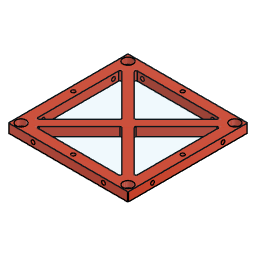
top-holder (Autodesk Fusion 360 design; units mm, degrees)
Autodesk Fusion 360 part; units mm, degrees
sketch "Sketch1" plane through (0, 0, 0) normal (0, 0, 1) x (1, 0, 0)
  line L0 (-44.9, 45) -> (49.5, 45)
  line L1 (49.8, 44.7) -> (49.8, -49.7)
  line L2 (49.5, -50) -> (-44.9, -50)
  line L3 (-45.2, -49.7) -> (-45.2, 44.7)
  arc A0 (-44.9, 45) -> (-45.2, 44.7) centre (-44.9, 44.7) ccw
  arc A1 (49.8, 44.7) -> (49.5, 45) centre (49.5, 44.7) ccw
  arc A2 (49.5, -50) -> (49.8, -49.7) centre (49.5, -49.7) ccw
  arc A3 (-45.2, -49.7) -> (-44.9, -50) centre (-44.9, -49.7) ccw
  point P0 (-45.2, 45)
  point P1 (49.8, 45)
  point P2 (-45.2, -50)
  dimension "d1" = 95
  dimension "d2" = 95
  dimension "d3" = 0.3
  dimension "d4" = 0.3
  constraint horizontal L0
  constraint vertical L1
  constraint horizontal L2
  constraint vertical L3
  constraint coincident P0 L0
  constraint coincident P0 L3
  constraint tangent L0 A0
  constraint tangent L3 A0
  constraint coincident P1 L0
  constraint coincident P1 L1
  constraint tangent L0 A1
  constraint tangent L1 A1
  constraint tangent L1 A2
  constraint tangent L2 A2
  constraint equal A1 A2
  constraint coincident P2 L2
  constraint coincident P2 L3
  constraint tangent L2 A3
  constraint tangent L3 A3
  constraint equal A1 A3
  measures "d1" distance of P0 P1
  measures "d2" distance of P0 P2
  measures "d3" radius of A0
  measures "d4" radius of A1
extrude "Extrude1" add sketch "Sketch1" along normal blind 7
sketch "Sketch2" plane through (0, 0, 7) normal (0, 0, 1) x (-1, 0, 0)
  arc A0 (44.9, -45) -> (45.2, -44.7) centre (44.9, -44.7) ccw
  line L0 (45.2, -44.7) -> (45.2, 49.7)
  arc A1 (45.2, 49.7) -> (44.9, 50) centre (44.9, 49.7) ccw
  line L1 (44.9, 50) -> (-49.5, 50)
  arc A2 (-49.5, 50) -> (-49.8, 49.7) centre (-49.5, 49.7) ccw
  line L2 (-49.8, 49.7) -> (-49.8, -44.7)
  arc A3 (-49.8, -44.7) -> (-49.5, -45) centre (-49.5, -44.7) ccw
  line L3 (-49.5, -45) -> (44.9, -45)
  line L4 (-38.8, 42) -> (34.2, 42)
  line L5 (37.2, 39) -> (37.2, -34)
  line L6 (34.2, -37) -> (-38.8, -37)
  line L7 (-41.8, -34) -> (-41.8, 39)
  arc A4 (-41.8, -34) -> (-38.8, -37) centre (-38.8, -34) ccw
  arc A5 (-38.8, 42) -> (-41.8, 39) centre (-38.8, 39) ccw
  arc A6 (37.2, 39) -> (34.2, 42) centre (34.2, 39) ccw
  arc A7 (34.2, -37) -> (37.2, -34) centre (34.2, -34) ccw
  point P0 (-41.8, 42)
  point P1 (37.2, 42)
  point P2 (-41.8, -37)
  dimension "d7" = 79
  dimension "d8" = 79
  dimension "d9" = 8
  dimension "d10" = 8
  dimension "d11" = 3
  constraint horizontal L4
  constraint vertical L5
  constraint horizontal L6
  constraint vertical L7
  constraint coincident P2 L6
  constraint coincident P2 L7
  constraint tangent L6 A4
  constraint tangent L7 A4
  constraint coincident P0 L4
  constraint coincident P0 L7
  constraint tangent L4 A5
  constraint tangent L7 A5
  constraint equal A4 A5
  constraint coincident P1 L4
  constraint coincident P1 L5
  constraint tangent L4 A6
  constraint tangent L5 A6
  constraint equal A4 A6
  constraint tangent L5 A7
  constraint tangent L6 A7
  constraint equal A4 A7
  measures "d7" distance of P0 P1
  measures "d8" distance of P0 P2
  measures "d9" distance of L1 L4
  measures "d10" distance of L2 L7
  measures "d11" radius of A4
extrude "Extrude2" cut sketch "Sketch2" against normal blind 10 contours L4 L5 L6 L7 A4 A5 A6 A7
sketch "Sketch3" plane through (0, 0, 7) normal (0, 0, 1) x (-1, 0, 0)
  line L0 (34.2, -37) -> (-38.8, -37)
  arc A0 (-41.8, -34) -> (-38.8, -37) centre (-38.8, -34) ccw
  line L1 (-41.8, -34) -> (-41.8, 39)
  arc A1 (-38.8, 42) -> (-41.8, 39) centre (-38.8, 39) ccw
  line L2 (-38.8, 42) -> (34.2, 42)
  arc A2 (37.2, 39) -> (34.2, 42) centre (34.2, 39) ccw
  line L3 (37.2, 39) -> (37.2, -34)
  arc A3 (34.2, -37) -> (37.2, -34) centre (34.2, -34) ccw
  arc A4 (44.9, -45) -> (45.2, -44.7) centre (44.9, -44.7) ccw
  line L4 (45.2, -44.7) -> (45.2, 49.7)
  arc A5 (45.2, 49.7) -> (44.9, 50) centre (44.9, 49.7) ccw
  line L5 (44.9, 50) -> (-49.5, 50)
  arc A6 (-49.5, 50) -> (-49.8, 49.7) centre (-49.5, 49.7) ccw
  line L6 (-49.8, 49.7) -> (-49.8, -44.7)
  arc A7 (-49.8, -44.7) -> (-49.5, -45) centre (-49.5, -44.7) ccw
  line L7 (-49.5, -45) -> (44.9, -45)
  line L8 (45.2, -45) -> (-49.75, 49.95)
sketch "Sketch4" plane through (0, 0, 7) normal (0, 0, 1) x (-1, 0, 0)
  line L0 (45.2, 50) -> (-49.8, -45)
sketch "Sketch5" plane through (0, 0, 7) normal (0, 0, 1) x (-1, 0, 0)
  line L0 (40.0749, -34.9251) -> (35.1251, -39.8749)
  line L1 (35.1251, -39.8749) -> (-45.1249, 40.3751)
  line L2 (-45.1249, 40.3751) -> (-40.1751, 45.3249)
  line L3 (-40.1751, 45.3249) -> (40.0749, -34.9251)
  line L4 (45.2, -45) -> (-49.75, 49.95)
  dimension "d14" = 3.5
  dimension "d15" = 3.5
  constraint perpendicular L0 L1
  constraint parallel L0 L2
  constraint parallel L1 L3
  measures "d14" distance of L1 L4
  measures "d15" distance of L3 L4
extrude "Extrude3" add sketch "Sketch5" against normal blind 7
sketch "Sketch6" plane through (0, 0, 7) normal (0, 0, 1) x (-1, 0, 0)
  line L0 (35.1251, 44.8749) -> (40.0749, 39.9251)
  line L1 (40.0749, 39.9251) -> (-41.1751, -41.3249)
  line L2 (-41.1751, -41.3249) -> (-46.1249, -36.3751)
  line L3 (-46.1249, -36.3751) -> (35.1251, 44.8749)
  line L4 (45.2, 50) -> (-49.8, -45)
  dimension "d18" = 3.5
  dimension "d19" = 3.5
  constraint perpendicular L0 L1
  constraint parallel L0 L2
  constraint parallel L1 L3
  measures "d18" distance of L3 L4
  measures "d19" distance of L1 L4
extrude "Extrude4" add sketch "Sketch6" against normal blind 7
sketch "Sketch7" plane through (0, 0, 7) normal (0, 0, 1) x (-1, 0, 0)
  line L0 (37.2, 37.0503) -> (37.2, -32.0503)
  line L1 (37.2, -32.0503) -> (2.6497, 2.5)
  line L2 (2.6497, 2.5) -> (37.2, 37.0503)
  line L3 (-2.3, -2.4497) -> (32.2503, -37)
  line L4 (32.2503, -37) -> (-36.8503, -37)
  line L5 (-36.8503, -37) -> (-2.3, -2.4497)
  line L6 (-7.2497, 2.5) -> (-41.8, -32.0503)
  line L7 (-41.8, -32.0503) -> (-41.8, 37.0503)
  line L8 (-41.8, 37.0503) -> (-7.2497, 2.5)
  line L9 (32.2503, 42) -> (-2.3, 7.4497)
  line L10 (-2.3, 7.4497) -> (-36.8503, 42)
  line L11 (-36.8503, 42) -> (32.2503, 42)
  arc A0 (44.9, -45) -> (45.2, -44.7) centre (44.9, -44.7) ccw
  line L12 (45.2, -44.7) -> (45.2, 49.7)
  arc A1 (45.2, 49.7) -> (44.9, 50) centre (44.9, 49.7) ccw
  line L13 (44.9, 50) -> (-49.5, 50)
  arc A2 (-49.5, 50) -> (-49.8, 49.7) centre (-49.5, 49.7) ccw
  line L14 (-49.8, 49.7) -> (-49.8, -44.7)
  arc A3 (-49.8, -44.7) -> (-49.5, -45) centre (-49.5, -44.7) ccw
  line L15 (-49.5, -45) -> (44.9, -45)
fillet "Fillet1" radius 1 1 edges at (36.8503, -42, 3.5)
fillet "Fillet2" radius 1 1 edges at (41.8, -37.0503, 3.5)
fillet "Fillet3" radius 1 1 edges at (41.8, 32.0503, 3.5)
fillet "Fillet4" radius 1 1 edges at (36.8503, 37, 3.5)
fillet "Fillet5" radius 1 1 edges at (-32.2503, 37, 3.5)
fillet "Fillet6" radius 1 1 edges at (-37.2, 32.0503, 3.5)
fillet "Fillet7" radius 1 1 edges at (-37.2, -37.0503, 3.5)
fillet "Fillet8" radius 1 1 edges at (-32.2503, -42, 3.5)
fillet "Fillet9" radius 1 1 edges at (-2.6497, -2.5, 3.5)
fillet "Fillet10" radius 1 1 edges at (2.3, -7.4497, 3.5)
fillet "Fillet11" radius 1 1 edges at (7.2497, -2.5, 3.5)
fillet "Fillet12" radius 1 1 edges at (2.3, 2.4497, 3.5)
sketch "Sketch8" plane through (0, 0, 7) normal (0, 0, 1) x (-1, 0, 0)
  line L0 (37.2, 34.636) -> (37.2, -29.636)
  arc A0 (35.4929, -30.3431) -> (37.2, -29.636) centre (36.2, -29.636) ccw
  line L1 (35.4929, -30.3431) -> (3.3569, 1.7929)
  arc A1 (3.3569, 3.2071) -> (3.3569, 1.7929) centre (4.064, 2.5) ccw
  line L2 (3.3569, 3.2071) -> (35.4929, 35.3431)
  arc A2 (37.2, 34.636) -> (35.4929, 35.3431) centre (36.2, 34.636) ccw
  arc A3 (29.836, -37) -> (30.5431, -35.2929) centre (29.836, -36) ccw
  line L3 (29.836, -37) -> (-34.436, -37)
  arc A4 (-35.1431, -35.2929) -> (-34.436, -37) centre (-34.436, -36) ccw
  line L4 (-35.1431, -35.2929) -> (-3.0071, -3.1569)
  arc A5 (-1.5929, -3.1569) -> (-3.0071, -3.1569) centre (-2.3, -3.864) ccw
  line L5 (-1.5929, -3.1569) -> (30.5431, -35.2929)
  line L6 (-41.8, -29.636) -> (-41.8, 34.636)
  arc A6 (-40.0929, 35.3431) -> (-41.8, 34.636) centre (-40.8, 34.636) ccw
  line L7 (-40.0929, 35.3431) -> (-7.9569, 3.2071)
  arc A7 (-7.9569, 1.7929) -> (-7.9569, 3.2071) centre (-8.664, 2.5) ccw
  line L8 (-7.9569, 1.7929) -> (-40.0929, -30.3431)
  arc A8 (-41.8, -29.636) -> (-40.0929, -30.3431) centre (-40.8, -29.636) ccw
  line L9 (-3.0071, 8.1569) -> (-35.1431, 40.2929)
  arc A9 (-34.436, 42) -> (-35.1431, 40.2929) centre (-34.436, 41) ccw
  line L10 (-34.436, 42) -> (29.836, 42)
  arc A10 (30.5431, 40.2929) -> (29.836, 42) centre (29.836, 41) ccw
  line L11 (30.5431, 40.2929) -> (-1.5929, 8.1569)
  arc A11 (-3.0071, 8.1569) -> (-1.5929, 8.1569) centre (-2.3, 8.864) ccw
  arc A12 (44.9, -45) -> (45.2, -44.7) centre (44.9, -44.7) ccw
  line L12 (45.2, -44.7) -> (45.2, 49.7)
  arc A13 (45.2, 49.7) -> (44.9, 50) centre (44.9, 49.7) ccw
  line L13 (44.9, 50) -> (-49.5, 50)
  arc A14 (-49.5, 50) -> (-49.8, 49.7) centre (-49.5, 49.7) ccw
  line L14 (-49.8, 49.7) -> (-49.8, -44.7)
  arc A15 (-49.8, -44.7) -> (-49.5, -45) centre (-49.5, -44.7) ccw
  line L15 (-49.5, -45) -> (44.9, -45)
  line L16 (44.9, 50) -> (-49.5, 50)
  line L17 (-49.5, -45) -> (44.9, -45)
  point P0 (40.2, 45)
  point P1 (-44.8, 45)
  point P2 (40.2, -40)
  point P3 (-44.8, -40)
  dimension "d46" = 5
  dimension "d47" = 5
  dimension "d48" = 5
  dimension "d49" = 5
  dimension "d50" = 5
  dimension "d51" = 5
  dimension "d52" = 5
  dimension "d53" = 5
  measures "d46" distance of P0 L16
  measures "d47" distance of L12 P0
  measures "d48" distance of P1 L16
  measures "d49" distance of L14 P1
  measures "d50" distance of L14 P3
  measures "d51" distance of P3 L17
  measures "d52" distance of P2 L17
  measures "d53" distance of L12 P2
hole "Hole1" at (44.8, 40, 7) at (-40.2, 40, 7) at (-40.2, -45, 7) at (44.8, -45, 7) direction (0, 0, -1) diameter 3 depth 15 tip angle 118
sketch "Sketch9" plane through (0, 0, 7) normal (0, 0, 1) x (-1, 0, 0)
  circle A0 centre (40.2, -40) radius 4
  line L0 (45.2, -44.7) -> (45.2, 49.7)
  line L1 (-49.5, -45) -> (44.9, -45)
  circle A1 centre (-44.8, -40) radius 4
  line L2 (-49.8, 49.7) -> (-49.8, -44.7)
  circle A2 centre (-44.8, 45) radius 4
  line L3 (44.9, 50) -> (-49.5, 50)
  circle A3 centre (40.2, 45) radius 4
  dimension "d57" = 8
  dimension "d58" = 5
  dimension "d59" = 5
  dimension "d60" = 8
  dimension "d61" = 5
  dimension "d62" = 5
  dimension "d63" = 8
  dimension "d64" = 5
  dimension "d65" = 5
  dimension "d66" = 8
  dimension "d67" = 5
  dimension "d68" = 5
  measures "d57" diameter of A0
  measures "d58" distance of A0.centre L0
  measures "d59" distance of A0.centre L1
  measures "d60" diameter of A1
  measures "d61" distance of A1.centre L2
  measures "d62" distance of L1 A1.centre
  measures "d63" diameter of A2
  measures "d64" distance of A2.centre L3
  measures "d65" distance of L2 A2.centre
  measures "d66" diameter of A3
  measures "d67" distance of L3 A3.centre
  measures "d68" distance of L0 A3.centre
extrude "Extrude5" cut sketch "Sketch9" against normal blind 5
sketch "Sketch10" plane through (0, 0, 7) normal (0, 0, 1) x (-1, 0, 0)
  line L0 (45.2, -44.7) -> (45.2, 49.7)
  line L1 (-49.5, -45) -> (44.9, -45)
  line L2 (-49.8, 49.7) -> (-49.8, -44.7)
  line L3 (44.9, 50) -> (-49.5, 50)
  point P0 (-2.3, -41)
  point P1 (41.2, 2.5)
  point P2 (-2.3, 46)
  point P3 (-45.8, 2.5)
  dimension "d71" = 4
  dimension "d72" = 47.5
  dimension "d73" = 4
  dimension "d74" = 47.5
  dimension "d75" = 4
  dimension "d76" = 47.5
  dimension "d77" = 4
  dimension "d78" = 47.5
  measures "d71" distance of P1 L0
  measures "d72" distance of P1 L1
  measures "d73" distance of P0 L1
  measures "d74" distance of P0 L2
  measures "d75" distance of P3 L2
  measures "d76" distance of P3 L3
  measures "d77" distance of P2 L3
  measures "d78" distance of P2 L0
hole "Hole2" at (2.3, -46, 7) at (-41.2, -2.5, 7) at (45.8, -2.5, 7) at (2.3, 41, 7) direction (0, 0, -1) diameter 3 depth 15 tip angle 118
sketch "Sketch11" plane through (0, -50, 0) normal (0, -1, 0) x (1, 0, 0)
  line L0 (-44.9, 0) -> (49.5, 0)
  line L1 (49.5, 0) -> (49.5, 7)
  line L2 (49.5, 7) -> (-44.9, 7)
  line L3 (-44.9, 7) -> (-44.9, 0)
  line L4 (49.8, 0) -> (49.8, 7)
  point P0 (-25.7, 3.5)
  point P1 (2.3, 3.5)
  point P2 (30.3, 3.5)
  dimension "d82" = 3.5
  dimension "d83" = 28
  dimension "d84" = 28
  dimension "d85" = 47.5
  dimension "d86" = 3.5
  dimension "d87" = 3.5
  measures "d82" distance of L0 P1
  measures "d83" horizontal distance of P0 P1
  measures "d84" horizontal distance of P1 P2
  measures "d85" distance of P1 L4
  measures "d86" distance of L0 P2
  measures "d87" distance of L0 P0
hole "Hole3" at (-25.7, -50, 3.5) at (30.3, -50, 3.5) direction (0, 1, 0) diameter 3 depth 11 tip angle 118
sketch "Sketch12" plane through (49.8, 0, 0) normal (1, 0, 0) x (0, 1, 0)
  line L0 (-49.7, 0) -> (44.7, 0)
  line L1 (44.7, 0) -> (44.7, 7)
  line L2 (44.7, 7) -> (-49.7, 7)
  line L3 (-49.7, 7) -> (-49.7, 0)
  line L4 (-50, 0) -> (-50, 7)
  point P0 (-30.5, 3.5)
  point P1 (-2.5, 3.5)
  point P2 (25.5, 3.5)
  dimension "d91" = 47.5
  dimension "d92" = 28
  dimension "d93" = 28
  dimension "d94" = 3.5
  dimension "d95" = 3.5
  dimension "d96" = 3.5
  measures "d91" distance of P1 L4
  measures "d92" distance of P0 P1
  measures "d93" distance of P1 P2
  measures "d94" distance of L0 P1
  measures "d95" distance of L0 P0
  measures "d96" distance of L0 P2
hole "Hole4" at (49.8, -30.5, 3.5) at (49.8, 25.5, 3.5) direction (-1, 0, 0) diameter 3 depth 11 tip angle 118
sketch "Sketch13" plane through (0, 0, 7) normal (0, 0, 1) x (1, 0, 0)
sketch "Sketch14" plane through (0, 45, 0) normal (0, 1, 0) x (-1, 0, 0)
  line L0 (-49.5, 0) -> (44.9, 0)
  line L1 (44.9, 0) -> (44.9, 7)
  line L2 (44.9, 7) -> (-49.5, 7)
  line L3 (-49.5, 7) -> (-49.5, 0)
  line L4 (-49.8, 0) -> (-49.8, 7)
  point P0 (-30.3, 3.5)
  point P1 (-2.3, 3.5)
  point P2 (25.7, 3.5)
  dimension "d100" = 47.5
  dimension "d101" = 28
  dimension "d102" = 28
  dimension "d103" = 3.5
  dimension "d104" = 3.5
  dimension "d105" = 3.5
  measures "d100" distance of P1 L4
  measures "d101" distance of P0 P1
  measures "d102" distance of P1 P2
  measures "d103" distance of L0 P1
  measures "d104" distance of L0 P2
  measures "d105" distance of L0 P0
hole "Hole5" at (30.3, 45, 3.5) at (-25.7, 45, 3.5) direction (0, -1, 0) diameter 3 depth 11 tip angle 118
sketch "Sketch15" plane through (-45.2, 0, 0) normal (-1, 0, 0) x (0, -1, 0)
  line L0 (-44.7, 0) -> (49.7, 0)
  line L1 (49.7, 0) -> (49.7, 7)
  line L2 (49.7, 7) -> (-44.7, 7)
  line L3 (-44.7, 7) -> (-44.7, 0)
  line L4 (-45, 0) -> (-45, 7)
  point P0 (-25.5, 3.5)
  point P1 (2.5, 3.5)
  point P2 (30.5, 3.5)
  dimension "d109" = 47.5
  dimension "d110" = 28
  dimension "d111" = 28
  dimension "d112" = 3.5
  dimension "d113" = 3.5
  dimension "d114" = 3.5
  measures "d109" distance of P1 L4
  measures "d110" distance of P0 P1
  measures "d111" distance of P1 P2
  measures "d112" distance of L0 P1
  measures "d113" distance of L0 P2
  measures "d114" distance of L0 P0
hole "Hole6" at (-45.2, 25.5, 3.5) at (-45.2, -30.5, 3.5) direction (1, 0, 0) diameter 3 depth 11 tip angle 118
